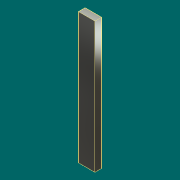
# Autodesk Inventor part: silvering
Saved by Autodesk Inventor 2016 SP1 (Build 200210100, 210)
## iProperties
Created: 2016-02-15
Part Number: silvering
Material: Silver
Document SubType Name: Modeling
Designer: sawai
Density: 10.49 g/cm^3
Appearance: Silver
Author: sawai
Autodesk Inventor part; units mm, degrees
ref_plane "YZ Plane" through (0, 0, 0) normal (1, 0, 0) x (0, 1, 0)
ref_plane "XZ Plane" through (0, 0, 0) normal (0, 1, 0) x (-1, 0, 0)
ref_plane "XY Plane" through (0, 0, 0) normal (0, 0, 1) x (1, 0, 0)
sketch "Sketch1" plane through (0, 0, 0) normal (0, 0, 1) x (1, 0, 0)
  line L0 (-12.5, 5) -> (12.5, 5)
  line L1 (12.5, 5) -> (12.5, -5)
  line L2 (12.5, -5) -> (-12.5, -5)
  line L3 (-12.5, -5) -> (-12.5, 5)
  line L4 (-12.5, 5) -> (12.5, -5) construction
  line L5 (12.5, 5) -> (-12.5, -5) construction
  line L6 (12.7, 5.2) -> (-12.7, 5.2)
  line L7 (-12.7, 5.2) -> (-12.7, -5.2)
  line L8 (-12.7, -5.2) -> (12.7, -5.2)
  line L9 (12.7, -5.2) -> (12.7, 5.2)
  point P0 (0, 0)
  dimension "d0" = 10
  dimension "d1" = 25
  dimension "d2" = 0.2
  constraints: 20 end point, 4 parallel, 2 midpoint, 2 perpendicular, 1 horizontal, 3 other
  measures "d0" distance of L0.end L1.end
  measures "d1" distance between parallel lines of L3 L1
  measures "d2" distance between parallel lines of L6 L0
extrude "Extrusion1" add sketch "Sketch1" along normal blind 200
sketch "Sketch2" plane through (0, 0, 200) normal (0, 0, 1) x (1, 0, 0)
  line L0 (12.7, 5.2) -> (-12.7, 5.2) projected
  line L1 (-12.7, 5.2) -> (-12.7, -5.2) projected
  line L2 (-12.7, -5.2) -> (12.7, -5.2) projected
  line L3 (12.7, -5.2) -> (12.7, 5.2) projected
  point P0 (0, 0)
extrude "Extrusion2" add sketch "Sketch2" along normal blind 0.2
equation "\"d0\" = ScintillatorThickness"
equation "\"d1\" = ScintillatorWidth"
equation "\"d2\" = silveringThickness"
equation "\"d3\" = ScintillatorHeight"
equation "\"d5\" = silveringThickness"
equation "\"ScintillatorThickness\" = 10"
equation "\"OpticalFiberClearence\" = 0.1"
equation "\"ScintillatorEdgeClearence\" = 3"
equation "\"ScintillatorWidth\" = 25"
equation "\"ScintillatorHeight\" = 200"
equation "\"ShallowTrackDepth\" = 1.2"
equation "\"DeepTrackDepth\" = 5.6"
equation "\"FiberEdgeOffsett\" = 5"
equation "\"LoopLargeTrackRatio\" = 1.1"
equation "\"FiberSensorClerence\" = 0.5"
equation "\"MountingScrewOffsett\" = 9"
equation "\"FoilThickness\" = 0.2"
equation "\"silveringThickness\" = 0.2"
body "Solid1"
